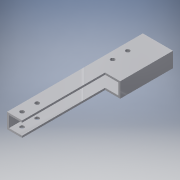
# Autodesk Inventor part: vertical support
Saved by Autodesk Inventor 2016 (Build 200138000, 138)
## iProperties
Created: 2016-02-06
Part Number: vertical support
Material: Aluminum 6061
Document SubType Name: Modeling
Designer: gus
Density: 2.7 g/cm^3
Appearance: Aluminum - Flat
Mass: 187.662 g
Surface Area: 460.951 cm^2
Volume: 69.5044 cm^3
Author: gus
Autodesk Inventor part; units mm, degrees
ref_plane "YZ Plane" through (0, 0, 0) normal (1, 0, 0) x (0, 1, 0)
ref_plane "XZ Plane" through (0, 0, 0) normal (0, 1, 0) x (-1, 0, 0)
ref_plane "XY Plane" through (0, 0, 0) normal (0, 0, 1) x (1, 0, 0)
sketch "Sketch1" plane through (0, 0, 0) normal (0, 0, 1) x (1, 0, 0)
  line L0 (0, 0) -> (-50.8, 0)
  line L1 (-50.8, 0) -> (-50.8, -25.4)
  line L2 (-50.8, -25.4) -> (0, -25.4)
  line L3 (0, -25.4) -> (0, 0)
  line L4 (-3.175, -22.225) -> (-47.625, -22.225)
  line L5 (-47.625, -22.225) -> (-47.625, -3.175)
  line L6 (-47.625, -3.175) -> (-3.175, -3.175)
  line L7 (-3.175, -3.175) -> (-3.175, -22.225)
  dimension "d0" = 50.8
  dimension "d1" = 25.4
  dimension "d2" = 3.175
  constraints: 16 end point, 4 parallel, 2 perpendicular, 1 horizontal, 3 other
  measures "d0" distance of L2.end L1.end
  measures "d1" distance of L1.end L0.end
  measures "d2" distance between parallel lines of L2 L4
extrude "Extrusion1" add sketch "Sketch1" along normal blind 228.6
sketch "Sketch2" plane through (-50.8, -25.4, 0) normal (0, -1, 0) x (1, 0, 0)
  line L0 (0, 228.6) -> (50.8, 228.6) projected
  line L1 (50.8, 228.6) -> (25.4, 228.6)
  line L2 (25.4, 228.6) -> (25.4, 88.9)
  line L3 (25.4, 88.9) -> (50.8, 88.9)
  line L4 (50.8, 88.9) -> (50.8, 228.6)
  point P0 (50.8, 0)
  dimension "d5" = 25.4
  dimension "d6" = 139.7
  constraints: 8 end point, 2 parallel, 1 horizontal, 1 perpendicular
  measures "d5" distance of L3.end L2.end
  measures "d6" distance of L2.end L1.end
extrude "Extrusion2" cut sketch "Sketch2" against normal blind 25.4
sketch "Sketch3" plane through (-50.8, -25.4, 0) normal (0, -1, 0) x (1, 0, 0)
  circle A0 centre (12.7, 215.9) radius 3.3734
  circle A1 centre (12.7, 190.5) radius 3.3734
  line L0 (25.4, 88.9) -> (25.4, 228.6) projected
  line L1 (0, 228.6) -> (25.4, 228.6) projected
  point P0 (50.8, 0)
  dimension "d9" = 6.7469
  dimension "d10" = 6.7469
  dimension "d11" = 12.7
  dimension "d12" = 12.7
  dimension "d13" = 12.7
  dimension "d14" = 38.1
  constraints: 2 centre point
  measures "d9" diameter of A0
  measures "d10" diameter of A1
  measures "d11" distance from line of L0 A1.centre
  measures "d12" distance from line of L0 A0.centre
  measures "d13" distance from line of L1 A0.centre
  measures "d14" distance from line of L1 A1.centre
extrude "Extrusion3" cut sketch "Sketch3" against normal blind 25.4
sketch "Sketch4" plane through (-50.8, 0, 0) normal (0, 1, 0) x (1, 0, 0)
  circle A0 centre (12.7, -50.8) radius 3.3734
  circle A1 centre (12.7, -76.2) radius 3.3782
  line L0 (50.8, 0) -> (0, 0) projected
  line L1 (0, 0) -> (0, -228.6) projected
  dimension "d17" = 6.7469
  dimension "d18" = 6.7564
  dimension "d19" = 50.8
  dimension "d20" = 12.7
  dimension "d21" = 12.7
  dimension "d22" = 25.4
  constraints: 2 centre point
  measures "d17" diameter of A0
  measures "d18" diameter of A1
  measures "d19" distance from line of L0 A0.centre
  measures "d20" distance from line of L1 A0.centre
  measures "d21" distance from line of L1 A1.centre
  measures "d22" distance of A0.centre A1.centre
extrude "Extrusion4" cut sketch "Sketch4" against normal blind 25.4
body "Solid1"
